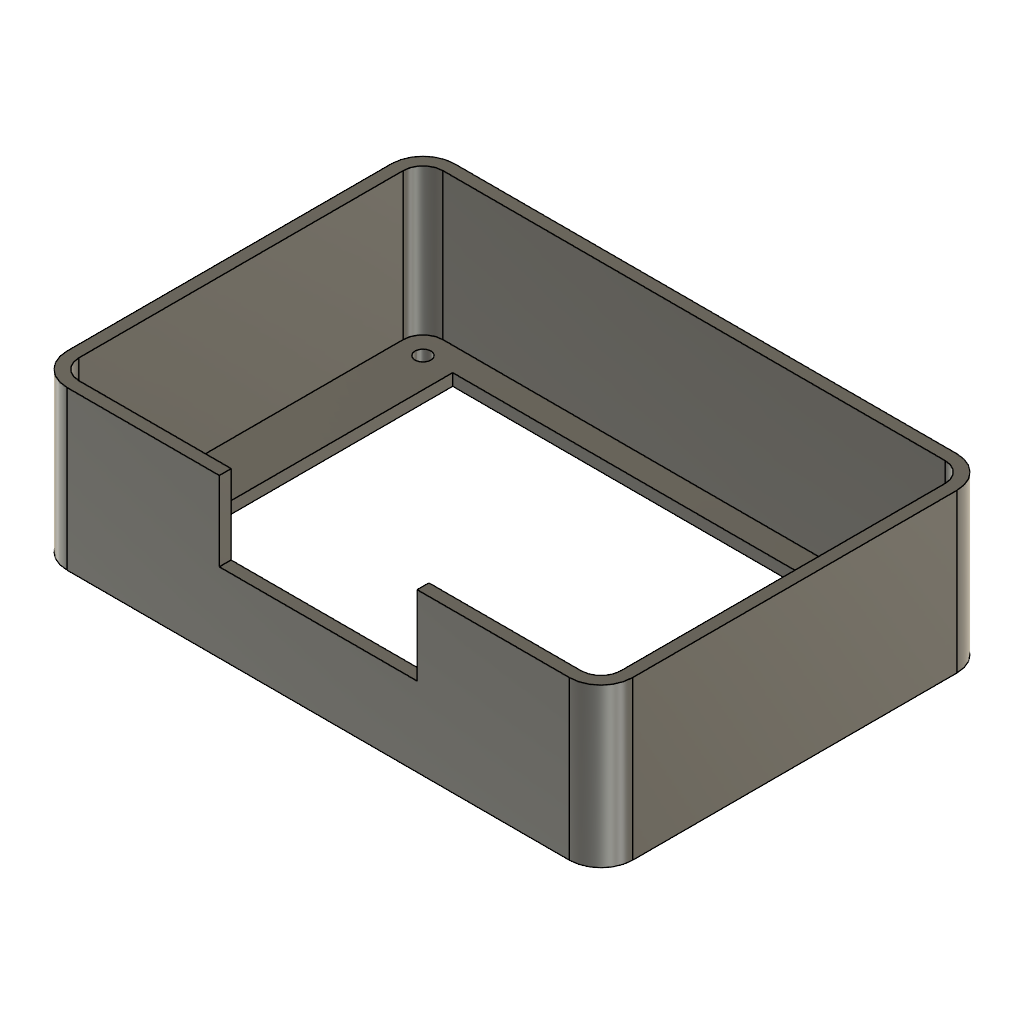
BASE_PCB (Autodesk Fusion 360 design; units mm, degrees)
Autodesk Fusion 360 part; units mm, degrees
sketch "Boceto1" plane through (0, 0, 0) normal (0, 0, 1) x (1, 0, 0)
  line L0 (-68.5, 46) -> (68.5, 46)
  line L1 (68.5, 46) -> (68.5, -46)
  line L2 (68.5, -46) -> (-68.5, -46)
  line L3 (-68.5, -46) -> (-68.5, 46)
  line L4 (-68.5, 46) -> (68.5, -46) construction
  line L5 (68.5, 46) -> (-68.5, -46) construction
  dimension "d1" = 137
  dimension "d2" = 92
  constraint horizontal L0
  constraint perpendicular L0 L1
  constraint parallel L0 L2
  constraint parallel L1 L3
  constraint coincident L4 origin
  constraint coincident L5 origin
  measures "d1" distance of L1.end L2.end
extrude "Extruir1" add sketch "Boceto1" along normal blind 3 makes body 1
sketch "Boceto2" plane through (0, 0, 3) normal (0, 0, 1) x (-1, 0, 0)
  line L0 (68.5, 46) -> (-68.5, 46)
  line L1 (-68.5, 46) -> (-68.5, -46)
  line L2 (-68.5, -46) -> (68.5, -46)
  line L3 (68.5, -46) -> (68.5, 46)
  line L4 (68.5, -46) -> (62.5, -46)
  line L5 (62.5, -46) -> (62.5, -40)
  line L6 (-68.5, -46) -> (-62.5, -46)
  line L7 (-62.5, -46) -> (-62.5, -40)
  line L8 (68.5, 46) -> (62.5, 46)
  line L9 (62.5, 46) -> (62.5, 40)
  line L10 (-68.5, 46) -> (-68.5, 40)
  line L11 (-68.5, 40) -> (-62.5, 40)
  circle A0 centre (62.5, -40) radius 2
  circle A1 centre (62.5, 40) radius 2
  circle A2 centre (-62.5, -40) radius 2
  circle A3 centre (-62.5, 40) radius 2
  dimension "d5" = 6
  dimension "d6" = 6
  dimension "d7" = 6
  dimension "d8" = 6
  dimension "d9" = 6
  dimension "d10" = 6
  dimension "d11" = 6
  dimension "d12" = 6
  dimension "d13" = 4
  dimension "d14" = 4
  dimension "d15" = 4
  dimension "d16" = 4
  constraint coincident L2.end L3.start
  constraint perpendicular L3 L4
  constraint perpendicular L4 L5
  constraint coincident L1.end L2.start
  constraint perpendicular L1 L6
  constraint perpendicular L6 L7
  constraint coincident L0.start L3.end
  constraint perpendicular L3 L8
  constraint perpendicular L8 L9
  constraint coincident L0.end L1.start
  constraint perpendicular L0 L10
  constraint perpendicular L1 L11
  constraint coincident L5.end A0.centre
  constraint coincident L9.end A1.centre
  constraint coincident L7.end A2.centre
  constraint coincident L11.end A3.centre
  measures "d13" diameter of A0
  measures "d14" diameter of A1
  measures "d15" diameter of A2
  measures "d16" diameter of A3
extrude "Extruir2" cut sketch "Boceto2" against normal blind 3 contours A0 | A1 | A2 | A3 bodies 1
fillet "Empalme1" radius 5 4 edges at (-68.5, -46, 1.5) (68.5, -46, 1.5) (68.5, 46, 1.5) (-68.5, 46, 1.5) on bodies 1
sketch "Boceto3" plane through (0, 0, 3) normal (0, 0, 1) x (-1, 0, 0)
  circle A0 centre (62.5, -40) radius 2
  circle A1 centre (-62.5, -40) radius 2
  circle A2 centre (62.5, 40) radius 2
  circle A3 centre (-62.5, 40) radius 2
  arc A4 (63.5, -46) -> (68.5, -41) centre (63.5, -41) ccw
  line L0 (68.5, -41) -> (68.5, 41)
  arc A5 (68.5, 41) -> (63.5, 46) centre (63.5, 41) ccw
  line L1 (63.5, 46) -> (-63.5, 46)
  arc A6 (-63.5, 46) -> (-68.5, 41) centre (-63.5, 41) ccw
  line L2 (-68.5, 41) -> (-68.5, -41)
  arc A7 (-68.5, -41) -> (-63.5, -46) centre (-63.5, -41) ccw
  line L3 (-63.5, -46) -> (63.5, -46)
  line L4 (-71.5, 41) -> (-71.5, -41)
  arc A8 (-71.5, -41) -> (-63.5, -49) centre (-63.5, -41) ccw
  line L5 (-63.5, -49) -> (63.5, -49)
  arc A9 (63.5, -49) -> (71.5, -41) centre (63.5, -41) ccw
  line L6 (71.5, -41) -> (71.5, 41)
  arc A10 (71.5, 41) -> (63.5, 49) centre (63.5, 41) ccw
  line L7 (63.5, 49) -> (-63.5, 49)
  arc A11 (-63.5, 49) -> (-71.5, 41) centre (-63.5, 41) ccw
  dimension "d21" = 3
extrude "Extruir3" add sketch "Boceto3" along normal blind 37 and the other way blind 3 separate body contours L4 A8 L5 A9 L6 A10 L7 A11 makes body 2
sketch "Boceto5" plane through (0, 0, 0) normal (0, 0, -1) x (1, 0, 0)
  arc A0 (-68.5, -41) -> (-63.5, -46) centre (-63.5, -41) ccw
  line L0 (-63.5, -46) -> (63.5, -46)
  arc A1 (63.5, -46) -> (68.5, -41) centre (63.5, -41) ccw
  line L1 (68.5, -41) -> (68.5, 41)
  arc A2 (68.5, 41) -> (63.5, 46) centre (63.5, 41) ccw
  line L2 (63.5, 46) -> (-63.5, 46)
  arc A3 (-63.5, 46) -> (-68.5, 41) centre (-63.5, 41) ccw
  line L3 (-68.5, 41) -> (-68.5, -41)
  circle A4 centre (-62.5, -40) radius 2
  circle A5 centre (62.5, -40) radius 2
  circle A6 centre (-62.5, 40) radius 2
  circle A7 centre (62.5, 40) radius 2
  line L4 (55, 40) -> (-55, 40)
  line L5 (-55, 40) -> (-55, -40)
  line L6 (-55, -40) -> (55, -40)
  line L7 (55, -40) -> (55, 40)
  line L8 (55, 40) -> (-55, -40) construction
  line L9 (-55, 40) -> (55, -40) construction
  dimension "d32" = 110
  dimension "d33" = 80
  constraint horizontal L4
  constraint perpendicular L4 L5
  constraint parallel L4 L6
  constraint parallel L5 L7
  constraint coincident L8 origin
  constraint coincident L9 origin
  measures "d32" distance of L5.end L6.end
  measures "d33" distance of L4.end L5.end
extrude "Extruir5" cut sketch "Boceto5" against normal blind 3 contours L4 L5 L6 L7 bodies 1
sketch "Boceto6" plane through (0, -49, 0) normal (0, -1, 0) x (1, 0, 0)
  line L0 (63.5, 0) -> (63.5, 40)
  line L1 (63.5, 40) -> (-63.5, 40)
  line L2 (-63.5, 40) -> (-63.5, 0)
  line L3 (-63.5, 0) -> (63.5, 0)
  line L4 (25, 40) -> (-25, 40)
  line L5 (-25, 40) -> (-25, 20)
  line L6 (-25, 20) -> (25, 20)
  line L7 (25, 20) -> (25, 40)
  point P0 (0, 40)
  dimension "d36" = 50
  constraint midpoint L4 P0
  constraint coincident L1 P0
  constraint perpendicular L0 L4
  constraint perpendicular L4 L5
  constraint perpendicular L5 L6
  constraint perpendicular L4 L7
  measures "d36" distance of L4.start L4.end
extrude "Extruir6" cut sketch "Boceto6" against normal blind 5 contours L1 L4 L5 L6 L7 bodies 2
